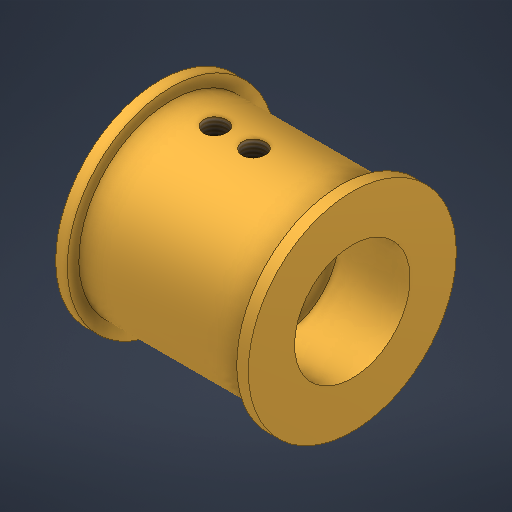
# Autodesk Inventor part: wheelGen2
Saved by Autodesk Inventor 2025 (Build 290162000, 162)
## iProperties
Created: 2025-03-26
Part Number: wheelGen2
Material: Mosaz, měkká žlutá
Document SubType Name: Modeling
Designer: Simak
Density: 8.47 g/cm^3
Appearance: Mosaz – satén
Mass: 82.776 g
Surface Area: 40.4389 cm^2
Volume: 9.77285 cm^3
Author: Simak
Autodesk Inventor part; units mm, degrees
ref_plane "YZ Plane" through (0, 0, 0) normal (1, 0, 0) x (0, 1, 0)
ref_plane "XY Plane" through (0, 0, 0) normal (0, 0, 1) x (1, 0, 0)
sketch "Náčrt1" plane through (0, 0, 0) normal (0, 0, 1) x (1, 0, 0)
  line L0 (0, 0) -> (25, 0)
  line L1 (0, 0) -> (0, 13.5)
  line L2 (0, 13.5) -> (1.5, 13.5)
  line L3 (1.5, 13.5) -> (1.5, 12)
  line L4 (1.5, 12) -> (23.5, 12)
  line L5 (23.5, 12) -> (23.5, 13.5)
  line L6 (23.5, 13.5) -> (25, 13.5)
  line L7 (25, 13.5) -> (25, 7.5)
  line L8 (25, 7.5) -> (15.75, 7.5)
  line L9 (48.5, 7.4) -> (48.5, -7.4) construction
  line L10 (6.5, 1.5) -> (6.5, -1.5) construction
  line L11 (15.75, 7.4) -> (15.75, -7.4) construction
  line L12 (6.5, 1.5) -> (15.75, 1.5) construction
  line L13 (6.5, -1.5) -> (15.75, -1.5) construction
  line L14 (15.75, 7.5) -> (15.75, 0)
  line L15 (13.75, 12) -> (13.75, 1.5) construction
  line L16 (10.75, 1.5) -> (10.75, 12) construction
  line L17 (8.75, 12) -> (8.75, 1.5) construction
  line L18 (5.75, 1.5) -> (5.75, 12) construction
  line L19 (15.75, 1.5) -> (0, 1.5)
  line L20 (5.75, 12) -> (7.25, 12) construction
  line L21 (7.25, 12) -> (8.75, 12) construction
  line L22 (12.25, 12) -> (10.75, 12) construction
  line L23 (12.25, 12) -> (13.75, 12) construction
  point P0 (6.5, 0)
  point P1 (24.25, 13.5)
  point P2 (15.75, 1.5)
  dimension "d1" = 15
  dimension "d2" = 48.5
  dimension "d3" = 42
  dimension "d4" = 3
  dimension "d5" = 9.25
  dimension "d6" = 14.8
  dimension "d7" = 27
  dimension "d8" = 25
  dimension "d9" = 1.5
  dimension "d10" = 1.5
  dimension "d11" = 3
  dimension "d12" = 2
  dimension "d13" = 3
  dimension "d14" = 2
  constraints: 46 end point, 18 point on line, 8 vertical, 7 perpendicular, 5 equal length, 3 midpoint, 2 horizontal alignment, 2 parallel, 1 horizontal, 11 other
  measures "d1" diameter of L8 L0
  measures "d2" distance between parallel lines of L1 L9
  measures "d3" distance between parallel lines of L9 L10
  measures "d4" distance of L10.start L10.end
  measures "d5" distance between parallel lines of L10 L11
  measures "d6" distance of L11.start L11.end
  measures "d7" diameter of point (24.25, 13.5) L0
  measures "d8" distance between parallel lines of L7 L1
  measures "d9" distance of L1.end L2.end
  measures "d10" distance of L2.end L3.end
  measures "d11" distance between parallel lines of L16 L15
  measures "d12" distance between parallel lines of L17 L16
  measures "d13" distance between parallel lines of L18 L17
  measures "d14" distance between parallel lines of L14 L15
revolve "Rotace1" add sketch "Náčrt1" angle 360 about axis through (0, 0, 0) along (1, 0, 0) contours L1 L2 L3 L4 L5 L6 L7 L8 L14 L19
ref_plane "Pracovní rovina1" through (12.5, 12, 0) normal (0, 1, 0) x (-1, 0, 0)
sketch "Náčrt2" plane through (12.5, 12, 0) normal (0, 1, 0) x (-1, 0, 0)
  point P0 (12.5, 0)
  point P1 (5.25, 0)
  point P2 (0.25, 0)
hole "Díra1" at (7.25, 12, 0) at (12.25, 12, 0) direction (0, -1, 0) diameter 3 depth 12
thread "Závit1" size "M3x0.5" class "6H" standard "ANSI Metric M Profile" full length
thread "Závit2" size "M3x0.5" class "6H" standard "ANSI Metric M Profile" full length
